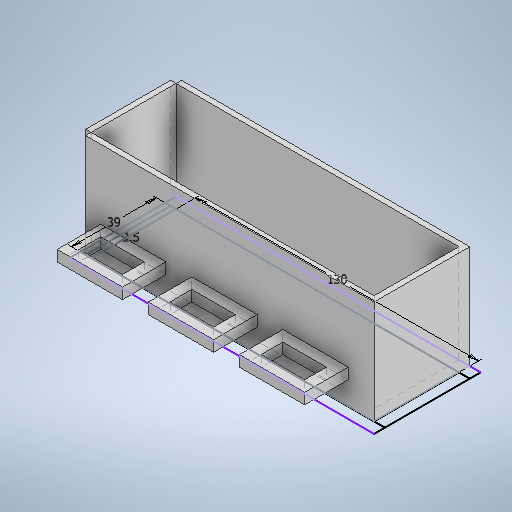
# Autodesk Inventor part: Part1
Saved by Autodesk Inventor 2025 (Build 290162010, 162A)
## iProperties
Created: 2024-07-08
Part Number: Part1
Material: Generic
Document SubType Name: Modeling
Designer: Dresden_Student
Density: 1 g/cm^3
Appearance: Default
Author: Dresden_Student
Autodesk Inventor part; units mm, degrees
ref_plane "YZ Plane" through (0, 0, 0) normal (1, 0, 0) x (0, 1, 0)
ref_plane "XZ Plane" through (0, 0, 0) normal (0, 1, 0) x (-1, 0, 0)
ref_plane "XY Plane" through (0, 0, 0) normal (0, 0, 1) x (1, 0, 0)
sketch "Sketch1" plane through (0, 0, 0) normal (0, 1, 0) x (-1, 0, 0)
  line L0 (0, 0) -> (130, 0)
  line L1 (130, 0) -> (130, -39)
  line L2 (130, -39) -> (0, -39)
  line L3 (0, -39) -> (0, 0)
  line L4 (0, -39) -> (-5, -39)
  line L5 (-5, -39) -> (-5, 0)
  line L6 (-5, 0) -> (0, 0)
  line L7 (0, 0) -> (0, -39)
  line L8 (130, -39) -> (135, -39)
  line L9 (135, -39) -> (135, 0)
  line L10 (135, 0) -> (130, 0)
  line L11 (130, 0) -> (130, -39)
  line L12 (-5, -39) -> (135, -39)
  line L13 (135, -39) -> (135, -44)
  line L14 (135, -44) -> (-5, -44)
  line L15 (-5, -44) -> (-5, -39)
  line L16 (135, 0) -> (-5, 0)
  line L17 (-5, 0) -> (-5, 5)
  line L18 (-5, 5) -> (135, 5)
  line L19 (135, 5) -> (135, 0)
  line L20 (130, -39) -> (130, 0)
  line L21 (132.5, -39) -> (132.5, 0)
  point P0 (132.5, -19.5)
  dimension "d0" = 130
  dimension "d1" = 39
  dimension "d55" = 2.5
  constraints: 44 end point, 10 parallel, 7 perpendicular, 5 horizontal, 4 collinear, 2 point on line, 2 vertical, 1 midpoint
  measures "d0" distance of L1.end L2.end
  measures "d1" distance of L0.end L1.end
  measures "d55" distance from line of L9 point (132.5, -19.5)
extrude "Extrusion1" add sketch "Sketch1" along normal blind 5 contours L0 L1 L2 L3
sketch "Sketch2" plane through (0, 5, 0) normal (0, 1, 0) x (1, 0, 0)
  point P0 (0, 0)
sketch "Sketch3" plane through (0, 5, 0) normal (0, 1, 0) x (1, 0, 0)
  point P0 (0, 0)
sketch "Sketch4" plane through (0, 5, 0) normal (0, 1, 0) x (1, 0, 0)
  point P0 (0, 0)
sketch "Sketch5" plane through (0, 5, 0) normal (0, 1, 0) x (1, 0, 0)
  point P0 (0, 0)
extrude "Extrusion2" add sketch "Sketch1" along normal blind 45 contours L6 L17 L18 L19 L10 L0 | L3 L4 L5 L6 | L2 L8 L13 L14 L15 L4
move faces "Move1" translate (0, 0, -2.5) faces at (-88.3333, 30, 5)
move faces "Move2" translate (0, 0, 2.5) faces at (-41.6667, 15, -44)
move faces "Move3" translate (-2.5, 0, 0) faces at (5, 15, -12.1667)
move faces "Move4" translate (0, 2.5, 0) faces at (-41.6667, 0, -13)
sketch "Sketch6" plane through (-135, 45, 2.5) normal (0, 0, 1) x (1, 0, 0)
  line L0 (95.625, -31.875) -> (125.625, -31.875)
  line L1 (125.625, -31.875) -> (125.625, -26.875)
  line L2 (125.625, -26.875) -> (95.625, -26.875)
  line L3 (95.625, -26.875) -> (95.625, -31.875)
  line L4 (0, -42.5) -> (137.5, -42.5) projected
  line L5 (0, 0) -> (137.5, 0) projected
  line L6 (53.75, -31.875) -> (83.75, -31.875)
  line L7 (83.75, -31.875) -> (83.75, -26.875)
  line L8 (83.75, -26.875) -> (53.75, -26.875)
  line L9 (53.75, -26.875) -> (53.75, -31.875)
  line L10 (11.875, -31.875) -> (41.875, -31.875)
  line L11 (41.875, -31.875) -> (41.875, -26.875)
  line L12 (41.875, -26.875) -> (11.875, -26.875)
  line L13 (11.875, -26.875) -> (11.875, -31.875)
  line L14 (0, -42.5) -> (0, 0) projected
  line L15 (137.5, -42.5) -> (137.5, 0) projected
  point P0 (135, -45)
  point P1 (11.875, -29.375)
  point P2 (53.75, -29.375)
  point P3 (41.875, -29.375)
  point P4 (95.625, -29.375)
  point P5 (83.75, -29.375)
  point P6 (125.625, -29.375)
  dimension "d18" = 30
  dimension "d19" = 5
  dimension "d20" = 10.625
  dimension "d27" = 42.5
  dimension "d28" = 30
  dimension "d29" = 5
  dimension "d30" = 30
  dimension "d31" = 5
  dimension "d32" = 11.875
  dimension "d33" = 11.875
  dimension "d34" = 11.875
  dimension "d35" = 137.5
  dimension "d36" = 11.875
  constraints: 24 end point, 6 midpoint, 6 parallel, 3 horizontal, 3 perpendicular
  measures "d18" distance of L0.start L0.end
  measures "d19" distance of L2.end L0.start
  measures "d20" distance between parallel lines of L0 L4
  measures "d27" distance between parallel lines of L4 L5
  measures "d28" distance of L6.start L6.end
  measures "d29" distance of L8.end L6.start
  measures "d30" distance of L10.start L10.end
  measures "d31" distance of L12.end L10.start
  measures "d32" distance from line of L14 point (11.875, -29.375)
  measures "d33" distance of point (53.75, -29.375) point (41.875, -29.375)
  measures "d34" distance of point (95.625, -29.375) point (83.75, -29.375)
  measures "d35" distance between parallel lines of L15 L14
  measures "d36" distance from line of L15 point (125.625, -29.375)
move faces "Move5" translate (5, 0, 0) faces at (-135, 16.6667, 0.8333) (-135, 16.6667, -40.6667)
move faces "Move6" translate (0, 5, 0) faces at (-42.5, 45, 1.6667)
extrude "Extrusion3" add sketch "Sketch6" along normal blind 30 contours L3 L2 L1 L0 | L9 L8 L7 L6 | L13 L12 L11 L10
move faces "Move7" translate (0, 0, -10) faces at (-103.125, 14.7917, 32.5) (-61.25, 16.4583, 32.5) (-19.375, 16.4583, 32.5)
sketch "Sketch7" plane through (-39.375, 18.125, 2.5) normal (0, 1, 0) x (1, 0, 0)
  line L0 (-78.75, -5) -> (-58.75, -5)
  line L1 (-58.75, -5) -> (-58.75, -15)
  line L2 (-58.75, -15) -> (-78.75, -15)
  line L3 (-78.75, -15) -> (-78.75, -5)
  line L4 (-53.75, 0) -> (-53.75, -20) projected
  line L5 (-83.75, 0) -> (-83.75, -20) projected
  line L6 (-53.75, -20) -> (-83.75, -20) projected
  line L7 (-90.625, 0) -> (41.875, 0) projected
  line L8 (-41.875, 0) -> (-41.875, -20) projected
  line L9 (-36.875, -5) -> (-16.875, -5)
  line L10 (-16.875, -5) -> (-16.875, -15)
  line L11 (-16.875, -15) -> (-36.875, -15)
  line L12 (-36.875, -15) -> (-36.875, -5)
  line L13 (5, -5) -> (25, -5)
  line L14 (25, -5) -> (25, -15)
  line L15 (25, -15) -> (5, -15)
  line L16 (5, -15) -> (5, -5)
  point P0 (39.375, 2.5)
  dimension "d42" = 5
  dimension "d43" = 20
  dimension "d44" = 10
  dimension "d45" = 30
  dimension "d46" = 20
  dimension "d47" = 5
  dimension "d48" = 41.875
  dimension "d49" = 20
  dimension "d50" = 10
  dimension "d51" = 20
  dimension "d52" = 10
  constraints: 24 end point, 6 parallel, 3 horizontal, 3 perpendicular
  measures "d42" distance between parallel lines of L4 L1
  measures "d43" distance of L0.start L0.end
  measures "d44" distance of L2.end L0.start
  measures "d45" distance between parallel lines of L4 L5
  measures "d46" distance between parallel lines of L6 L7
  measures "d47" distance between parallel lines of L0 L7
  measures "d48" distance between parallel lines of L8 L5
  measures "d49" distance of L9.start L10.start
  measures "d50" distance of L11.end L9.start
  measures "d51" distance of L13.start L14.start
  measures "d52" distance of L15.end L13.start
extrude "Extrusion4" cut sketch "Sketch7" against normal blind 30 contours L0 L1 L2 L3 | L9 L10 L11 L12 | L13 L14 L15 L16
extrude "Extrusion5" add sketch "Sketch1" along normal up to surface (50 mm away) contours L10 L21 L8 L1
move faces "Move8" translate (0, 2.5, 0) faces at (-131.6667, 0, -26)
equation "\"d18\" = d30"
equation "\"d20\" = 0.25 * d27"
equation "\"d28\" = d30"
equation "\"d32\" = -0.75 * d30 + 0.25 * d35"
equation "\"d33\" = -0.75 * d30 + 0.25 * d35"
equation "\"d34\" = -0.75 * d30 + 0.25 * d35"
equation "\"d36\" = -0.75 * d30 + 0.25 * d35"
equation "\"d42\" = -0.5 * d43 + 0.5 * d45"
equation "\"d47\" = -0.5 * d44 + 0.5 * d46"
body "Solid1"
